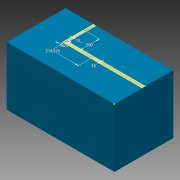
# Autodesk Inventor part: River 3_赤
Saved by Autodesk Inventor 2015 (Build 190159000, 159)
## iProperties
Created: 2015-08-24
Part Number: River 3_赤
Material: 一般
Document SubType Name: Modeling
Designer: nobuhiro
Density: 1 g/cm^3
Appearance: スカイ ブルー 標準
Author: nobuhiro
Autodesk Inventor part; units mm, degrees
ref_plane "YZ Plane" through (0, 0, 0) normal (1, 0, 0) x (0, 1, 0)
ref_plane "XZ Plane" through (0, 0, 0) normal (0, 1, 0) x (-1, 0, 0)
ref_plane "XY Plane" through (0, 0, 0) normal (0, 0, 1) x (1, 0, 0)
sketch "スケッチ1" plane through (0, 0, 0) normal (0, 0, 1) x (1, 0, 0)
  line L0 (0, 0) -> (-1100, 0)
  line L1 (-1100, 0) -> (-1100, 600)
  line L2 (-1100, 600) -> (0, 600)
  line L3 (0, 600) -> (0, 0)
  line L4 (-815, 600) -> (-785, 600)
  line L5 (-785, 600) -> (-785, 285)
  line L6 (-785, 285) -> (-815, 285)
  line L7 (-815, 285) -> (-815, 600)
  line L8 (-815, 285) -> (0, 285)
  line L9 (0, 285) -> (0, 315)
  line L10 (0, 315) -> (-815, 315)
  line L11 (-815, 315) -> (-815, 285)
  point P0 (0, 300)
  point P1 (0, 300)
  dimension "d0" = 1100
  dimension "d1" = 600
  dimension "d2" = 30
  dimension "d3" = 785
  constraints: 24 end point, 6 parallel, 4 perpendicular, 3 horizontal, 2 midpoint, 2 point on line, 1 coincident
  measures "d0" distance of L1.end L2.end
  measures "d1" distance of L0.end L1.end
  measures "d2" distance between parallel lines of L8 L10
  measures "d3" distance between parallel lines of L3 L5
extrude "押し出し1" add sketch "スケッチ1" along normal blind 600 contours L0 L1 L2 L7 L6 L8 L3 | L10 L5 L2 L3
sketch "スケッチ2" plane through (0, 0, 0) normal (0, 0, -1) x (-1, 0, 0)
  line L0 (815, 285) -> (0, 285) projected
  line L1 (815, 600) -> (815, 285) projected
  line L2 (0, 315) -> (785, 315) projected
  line L3 (785, 315) -> (785, 600) projected
  line L4 (0, 600) -> (785, 600) projected
  line L5 (0, 315) -> (0, 600) projected
  line L6 (815, 600) -> (785, 600)
  line L7 (0, 315) -> (0, 285)
  constraints: 4 end point, 1 horizontal, 1 perpendicular
extrude "押し出し2" add sketch "スケッチ2" against normal blind 600.1 contours L0 L7 L2 L3 L6 L1
sketch "スケッチ3" plane through (0, 0, 600.1) normal (0, 0, 1) x (1, 0, 0)
  line L0 (-815, 600) -> (-815, 285) projected
  line L1 (-815, 285) -> (0, 285) projected
  line L2 (0, 315) -> (-785, 315) projected
  point P0 (0, 0)
  point P1 (-800, 300)
  point P2 (-800, 500)
  point P3 (-400, 300)
  dimension "d8" = 15
  dimension "d9" = 15
  dimension "d10" = 15
  dimension "d11" = 200
  dimension "d12" = 400
  dimension "d13" = 15
  measures "d8" distance from line of point (-800, 300) L0
  measures "d9" distance from line of point (-800, 300) L1
  measures "d10" distance from line of L0 point (-800, 500)
  measures "d11" distance of point (-800, 300) point (-800, 500)
  measures "d12" distance of point (-800, 300) point (-400, 300)
  measures "d13" distance from line of L2 point (-400, 300)
equation "\"d9\" = d8"
